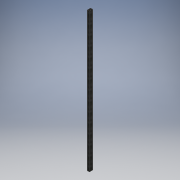
# Autodesk Inventor part: 2570 STEEL PROFILE 60X40X2
Saved by Autodesk Inventor 2018 (Build 220112000, 112)
## iProperties
Created: 2018-10-15
Part Number: 2570 STEEL PROFILE 60X40X2
Material: Acero
Document SubType Name: Modeling
Designer: Toshiba
Density: 7.85 g/cm^3
Appearance: Placa
Author: Toshiba
Autodesk Inventor part; units mm, degrees
ref_plane "YZ Plane" through (0, 0, 0) normal (1, 0, 0) x (0, 1, 0)
ref_plane "XZ Plane" through (0, 0, 0) normal (0, 1, 0) x (-1, 0, 0)
ref_plane "XY Plane" through (0, 0, 0) normal (0, 0, 1) x (1, 0, 0)
sketch "Boceto1" plane through (0, 0, 0) normal (0, 0, 1) x (1, 0, 0)
  line L0 (20, -30) -> (20, 30)
  line L1 (20, 30) -> (-20, 30)
  line L2 (-20, 30) -> (-20, -30)
  line L3 (-20, -30) -> (20, -30)
  line L4 (20, -30) -> (-20, 30) construction
  line L5 (20, 30) -> (-20, -30) construction
  line L6 (-18, -28) -> (-18, 28)
  line L7 (-18, 28) -> (18, 28)
  line L8 (18, 28) -> (18, -28)
  line L9 (18, -28) -> (-18, -28)
  point P0 (0, 0)
  dimension "d0" = 60
  dimension "d1" = 40
  dimension "d2" = 2
  constraints: 20 end point, 4 parallel, 2 midpoint, 2 perpendicular, 1 vertical, 3 other
  measures "d0" distance of L0.start L0.end
  measures "d1" distance of L1.end L0.end
  measures "d2" distance between parallel lines of L2 L6
extrude "Extrusión1" add sketch "Boceto1" along normal mid plane 2570
sketch "Boceto2" plane through (-20, 30, 1285) normal (0, 1, 0) x (1, 0, 0)
  circle A0 centre (20, 214) radius 5
  line L0 (40, 0) -> (0, 0) projected
  circle A1 centre (20, 428) radius 5
  circle A2 centre (20, 642) radius 5
  circle A3 centre (20, 856) radius 5
  circle A4 centre (20, 1070) radius 5
  line L1 (-137.4788, 1285) -> (186.1246, 1285)
  circle A5 centre (20, 2356) radius 5
  circle A6 centre (20, 2142) radius 5
  circle A7 centre (20, 1928) radius 5
  circle A8 centre (20, 1714) radius 5
  circle A9 centre (20, 1500) radius 5
  point P0 (20, 1285)
  dimension "d5" = 10
  dimension "d6" = 214
  dimension "d9" = 10
  dimension "d10" = 214
  dimension "d11" = 10
  dimension "d12" = 214
  dimension "d13" = 10
  dimension "d14" = 214
  dimension "d15" = 10
  dimension "d16" = 214
  dimension "d17" = 215
  constraints: 10 centre point, 5 symmetric about line, 2 end point, 1 horizontal, 5 other
  measures "d5" diameter of A0
  measures "d6" distance from line of L0 A0.centre
  measures "d9" diameter of A1
  measures "d10" distance of A0.centre A1.centre
  measures "d11" diameter of A2
  measures "d12" distance of A1.centre A2.centre
  measures "d13" diameter of A3
  measures "d14" distance of A2.centre A3.centre
  measures "d15" diameter of A4
  measures "d16" distance of A3.centre A4.centre
  measures "d17" distance from line of L1 A4.centre
extrude "Extrusión3" cut sketch "Boceto2" against normal blind 2
